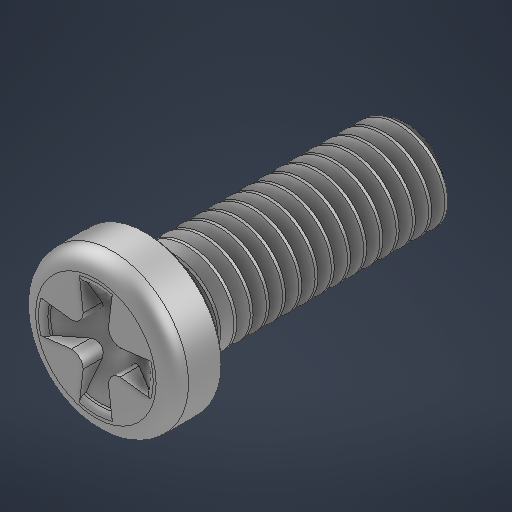
# Autodesk Inventor part: M5 x0.8ALT (...)_L11
Saved by Autodesk Inventor 2025.2 (Build 292293000, 293)
## iProperties
Created: 2024-12-01
Part Number: M5 x0.8ALT (...)_L11
Material: Generic
Document SubType Name: Modeling
Designer: Tiago
Density: 1 g/cm^3
Appearance: Anodized - Light Gray
Author: Tiago
Autodesk Inventor part; units mm, degrees
ref_plane "YZ Plane" through (0, 0, 0) normal (1, 0, 0) x (0, 1, 0)
ref_plane "XZ Plane" through (0, 0, 0) normal (0, 1, 0) x (-1, 0, 0)
sketch "Sketch2" plane through (0, 0, 0) normal (0, 1, 0) x (-1, 0, 0)
  line L0 (0, -1.5) -> (0, -13.6)
  line L1 (-1.3865, -13.6) -> (-1.3865, -2.2)
  line L2 (-3.3, 0) -> (-2.3, 0)
  line L3 (-2.1902, -0.2355) -> (0, -1.5)
  line L4 (-2.3, 0) -> (-2.1902, -0.2355)
  line L5 (-3.3, 0) -> (-3.3, -2.2)
  line L6 (-3.3, -2.2) -> (-1.3865, -2.2)
  line L7 (-1.3865, -13.6) -> (0, -13.6)
  line L8 (0, -13.6) -> (-2, -13.6)
  line L9 (-2, -13.6) -> (-2, -15.5311)
  line L10 (-2, -15.5311) -> (0, -15.5311)
  line L11 (0, -15.5311) -> (0, -13.6)
  line L12 (-2, -13.6) -> (-2, -11.1)
  line L13 (-1.3865, -13.6) -> (-2, -13.2458)
  point P0 (0, 0)
  point P1 (-2.8, 0)
  point P2 (0, -11.7)
  point P3 (-2, -12.508)
  dimension "d0" = 2.773
  dimension "d3" = 4.6
  dimension "d4" = 60
  dimension "d5" = 25
  dimension "d6" = 1.5
  dimension "k" = 2.2
  dimension "L" = 13.6
  dimension "d79" = 6.6
  dimension "d84" = 4
  dimension "d91" = 30
  constraints: 28 end point, 5 point on line, 3 parallel, 3 vertical, 2 horizontal, 2 horizontal alignment, 2 perpendicular, 1 midpoint
  measures "d0" diameter of L1 L0
  measures "d3" diameter of L2.end L0
  measures "d4" angle of L3 L0
  measures "d5" angle of L0 L4
  measures "d6" vertical distance of L0.start point (-2.8, 0)
  measures "k" vertical distance of L1.end L2.start
  measures "L" distance from line of L0.end L2
  measures "d79" diameter of L2.start L0
  measures "d84" diameter of L9 L0
  measures "d91" angle of L8 L13
revolve "Revolution1" add sketch "Sketch2" angle 360 about axis through (0, 0, -1.5) along (0, 0, -1) contours L0 L7 L1 L6 L5 L2 L4 L3
sketch "Sketch3" plane through (0, 0, 0) normal (0, 0, 1) x (1, 0, 0)
  line L0 (0, 4.62) -> (0, -4.62) projected
  line L1 (-4.7426, 0) -> (5.3553, 0) projected
  circle A0 centre (0, 0) radius 2.3 projected
  line L2 (0, 2.3) -> (0.6965, 2.3) construction
  line L3 (0, 2.3) -> (-0.697, 2.3)
  line L4 (2.3, 0) -> (2.3, 0.6965) construction
  line L5 (2.3, 0) -> (2.3, -0.6965) construction
  line L6 (-0.697, 2.3) -> (-0.697, 2.1918)
  line L7 (0.6965, 2.3) -> (0.6965, 2.192)
  line L8 (2.192, 0.6965) -> (2.3, 0.6965)
  arc A1 (2.3, 0.6965) -> (0.6965, 2.3) centre (0, 0) ccw
  line L9 (-0.697, -0.0285) -> (-0.697, 0.3205) construction
  line L10 (-0.5455, 1.0455) -> (0.5455, 1.0455) construction
  line L11 (-0.697, 2.3) -> (-0.5455, 1.0455)
  line L12 (0.6965, 2.3) -> (0.5455, 1.0455)
  line L13 (0.6965, 0.6965) -> (1.0455, 0.6965) construction
  line L14 (1.0455, -0.5455) -> (1.0455, 0.5455) construction
  line L15 (1.0455, 0.5455) -> (2.3, 0.6965)
  line L16 (1.0455, -0.5455) -> (2.3, -0.6965)
  line L17 (0.6965, 0.6965) -> (0.6965, 1.0455) construction
  arc A2 (0.5455, 1.0455) -> (1.0455, 0.5455) centre (1.0617, 1.0617) ccw
  line L18 (-2.3, 0) -> (-2.3, 0.6965) construction
  arc A3 (-0.6965, 2.3) -> (-2.3, 0.6965) centre (0, 0) ccw
  line L19 (-1.0455, 0.5455) -> (-2.3, 0.6965)
  arc A4 (-1.0455, 0.5455) -> (-0.5455, 1.0455) centre (-1.0617, 1.0617) ccw
  line L20 (0, -2.3) -> (0.6965, -2.3) construction
  line L21 (0, -2.3) -> (-0.697, -2.3) construction
  line L22 (-0.697, -2.3) -> (-0.5455, -1.0455)
  line L23 (0.6965, -2.3) -> (0.5455, -1.0455)
  arc A5 (1.0455, -0.5455) -> (0.5455, -1.0455) centre (1.0617, -1.0617) ccw
  arc A6 (-0.5455, -1.0455) -> (-1.0455, -0.5455) centre (-1.0617, -1.0617) ccw
  line L24 (-2.3, 0) -> (-2.3, -0.6965) construction
  line L25 (-1.0455, -0.5455) -> (-2.3, -0.6965)
  arc A7 (-2.3, -0.6965) -> (-0.697, -2.3) centre (0.5455, 0.5451) ccw
  arc A8 (0.6965, -2.3) -> (3.5708, -0.1516) centre (0.6175, 0.8027) ccw
  point P0 (0, 0)
  point P1 (0, 1.0455)
  point P2 (1.0455, 0)
  point P3 (-2.1959, -0.684)
  point P4 (-0.6844, -2.1958)
  point P5 (-0.6844, 2.1958)
  point P6 (-2.1959, 0.684)
  point P7 (0.684, -2.1959)
  point P8 (2.1959, -0.684)
  point P9 (2.1959, 0.684)
  point P10 (0.684, 2.1959)
  dimension "d12" = 0.6965
  dimension "d13" = 0.697
  dimension "d14" = 0.6965
  dimension "d15" = 0.6965
  dimension "d17" = 0.349
  dimension "d20" = 1.091
  dimension "d21" = 0.349
  dimension "d22" = 1.091
  constraints: 48 end point, 23 point on circle, 14 symmetric about line, 8 centre point, 6 point on line, 4 horizontal, 4 vertical, 2 midpoint, 2 perpendicular, 2 tangent, 4 other
  measures "d12" distance of L2.start L2.end
  measures "d13" distance of L2.start L3.end
  measures "d14" distance of L4.start L4.end
  measures "d15" distance of L4.start L5.end
  measures "d17" distance of L9.start L9.end
  measures "d20" distance of L10.start L10.end
  measures "d21" distance of L13.start L13.end
  measures "d22" distance of L14.start L14.end
extrude "Extrusion1" add sketch "Sketch3" against normal up to next contours A0 L15 A2 L12 | L11 A4 L19 A0 | A0 L25 A6 L22 | L23 A5 L16 A0
fillet "Fillet1" radius 0.274 4 edges at (-0.0002, 2.3, 0) (2.3, 0, 0) (-0.0002, -2.3, 0) (-2.3, 0, 0)
sketch "Sketch4" plane through (0, 0, 0) normal (0, 1, 0) x (-1, 0, 0)
  line L0 (0, -17.9273) -> (0, 3.0301) projected
  line L1 (-2, -14.4542) -> (-2, -14.5792)
  line L2 (-2, -14.5792) -> (-1.3865, -14.9334)
  line L3 (-1.3865, -14.9334) -> (-1.3865, -14.1)
  line L4 (-2, -14.4542) -> (-1.3865, -14.1)
  line L5 (-2, -14.5167) -> (-1.3865, -14.5167)
  line L6 (0, -10) -> (0, -9)
  line L7 (2.1429, -9) -> (-2.1429, -9)
  line L8 (-1.3865, -2.2) -> (-3.3, -2.2) projected
  line L9 (-3.3, -2.2) -> (-3.3, 0) projected
  line L10 (3.3, 0) -> (3.3, -2.2) projected
  line L11 (3.3, -2.2) -> (1.3865, -2.2) projected
  line L12 (-3.3, 0) -> (-2.4746, 0) projected
  line L13 (-2.1902, -0.2355) -> (0, -1.5) projected
  line L14 (0, -1.5) -> (2.1902, -0.2355) projected
  line L15 (2.4746, 0) -> (3.3, 0) projected
  line L16 (1.3865, -2.2) -> (1.3865, -13.6) projected
  line L17 (-1.3865, -13.6) -> (-1.3865, -2.2) projected
  line L18 (1.3865, -13.6) -> (-1.3865, -13.6) projected
  arc A0 (-2.2262, -0.1582) -> (-2.4746, 0) centre (-2.4746, -0.274) ccw projected
  line L19 (-2.2262, -0.1582) -> (-2.1902, -0.2355) projected
  line L20 (2.1902, -0.2355) -> (2.2262, -0.1582) projected
  arc A1 (2.4746, 0) -> (2.2262, -0.1582) centre (2.4746, -0.274) ccw projected
  point P0 (0, 0)
  point P1 (-2, -13.9542)
  point P2 (0, -10.9667)
  dimension "d" = 2.773
  dimension "d28" = 0.5
  dimension "d77" = 0.125
  dimension "d78" = 60
  dimension "d81" = 0.5
  dimension "d90" = 0.6135
  constraints: 14 end point, 3 midpoint, 3 point on line, 2 horizontal, 1 equal length, 1 parallel, 1 vertical
  measures "d" diameter of L3 L0
  measures "d28" distance of point (-2, -13.954) L1.start
  measures "d77" distance of L1.start L1.end
  measures "d78" angle of L2 L4
  measures "d81" distance of L17.start L3.end
  measures "d90" distance of L5.start L5.end
coil "Coil1" sketch "Sketch4" operation add axis through (0, 0, -10) along (0, 0, 1) pitch 0.7 turns 18 hand right contours L4 L3 L5 L1 | L5 L3 L2 L1
ref_plane "Work Plane1" through (0, 0, -3) normal (0, 0, 1) x (1, 0, 0)
chamfer "Chamfer5" distance 0.1 angle 45 1 edges at (-3.3, 0, -2.2)
fillet "Fillet3" radius 0.7 1 edges at (-3.3, 0, 0)
revolve "Revolution3" cut sketch "Sketch2" angle 360 about axis through (0, 0, -1.5) along (0, 0, -1) contours L11 L10 L9 L8 L7 | L8 L12 L13
equation "\"M\" = 4"
body "Solid1"
